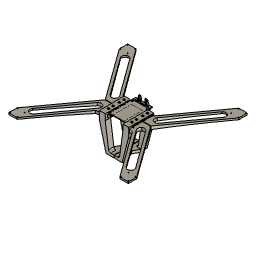
Drone Frame (Autodesk Fusion 360 design; units mm, degrees)
Autodesk Fusion 360 part; units mm, degrees
note: some values were not read from the file. Chosen so that the rebuilt part matches the saved one: a direction; which face or edge a step refers to. Set by a fixed rule: which sketch regions a step uses.
sketch "Sketch1" plane through (0, 0, 0) normal (0, 1, 0) x (1, 0, 0)
  line L0 (0, 0) -> (0, 2.5)
  line L1 (0, 0) -> (49.8, 0)
  line L2 (49.8, 0) -> (49.8, 2.5)
  line L3 (0, 2.5) -> (3, 2.5)
  line L4 (3, 2.5) -> (3, 7.5)
  line L5 (3, 7.5) -> (-2.5, 7.5)
  line L6 (-2.5, 7.5) -> (-2.5, -5)
  line L7 (-2.5, -5) -> (24.9, -5)
  line L8 (24.9, 0) -> (24.9, -5)
  line L9 (52.3, 7.5) -> (52.3, -5)
  line L10 (46.8, 7.5) -> (52.3, 7.5)
  line L11 (46.8, 2.5) -> (46.8, 7.5)
  line L12 (49.8, 2.5) -> (46.8, 2.5)
  line L13 (52.3, -5) -> (24.9, -5)
  dimension "d1" = 2.5
  dimension "d2" = 49.8
  dimension "d3" = 3
  dimension "d4" = 5
  dimension "d5" = 5
  dimension "d6" = 2.5
  constraint coincident L0.start L1.start
  constraint vertical L0
  constraint perpendicular L0 L1
  constraint perpendicular L1 L2
  constraint horizontal L0.end L2.end
  constraint perpendicular L0 L3
  constraint perpendicular L3 L4
  constraint perpendicular L4 L5
  constraint perpendicular L5 L6
  constraint perpendicular L6 L7
  constraint midpoint L1 L8.start
  constraint perpendicular L7 L8
  constraint symmetric L0.end L8 L2.end
  constraint symmetric L3.end L8 L11.start
  constraint symmetric L4.end L8 L10.start
  constraint symmetric L5.end L8 L9.start
  constraint symmetric L6.end L8 L9.end
  constraint symmetric L7.end L8 L13.end
  measures "d1" distance of L0.start L0.end
  measures "d2" distance of L0.start L1.end
  measures "d3" distance of L0.end L3.end
  measures "d4" distance of L3.end L4.end
  measures "d5" distance of L7.end L8.start
  measures "d6" distance of L0 L6
extrude "Extrude1" add sketch "Sketch1" along normal blind 65 makes body 1
sketch "Sketch2" plane through (0, 0, 0) normal (0, 0, -1) x (1, 0, 0)
  line L0 (49.8, 0) -> (0, 0)
  line L1 (0, 0) -> (0, -65)
  line L2 (0, -65) -> (49.8, -65)
  line L3 (49.8, -65) -> (49.8, 0)
  line L4 (49.8, -61) -> (0, -61)
  dimension "d9" = 4
  constraint coincident L3 L4.start
  constraint coincident L1 L4.end
  constraint perpendicular L1 L4
  measures "d9" distance of L2 L4
extrude "Extrude2" add sketch "Sketch2" along normal blind 4 contours L1 L2 L3 L4 bodies 1
sketch "Sketch3" plane through (0, 0, 0) normal (0, 0, -1) x (1, 0, 0)
  line L0 (0, -61) -> (49.8, -61)
  line L1 (49.8, -61) -> (49.8, 0)
  line L2 (49.8, 0) -> (0, 0)
  line L3 (0, 0) -> (0, -61)
  line L4 (3, 0) -> (3, -65)
  line L5 (46.8, 0) -> (46.8, -65)
  line L6 (46.8, -61) -> (3, -61)
  line L7 (0, 0) -> (49.8, 0)
  line L8 (3, -65) -> (46.8, -65)
  line L9 (46.8, -65) -> (46.8, 0)
  line L10 (46.8, 0) -> (3, 0)
  line L11 (3, 0) -> (3, -65)
  line L12 (3, -65) -> (3, -61)
  line L13 (46.8, -65) -> (46.8, -61)
  constraint horizontal L8
  constraint vertical L9
  constraint horizontal L10
  constraint vertical L11
  constraint coincident L5.start L9.end
  constraint coincident L4.end L8.start
extrude "Extrude3" cut sketch "Sketch3" against normal blind 5 contours L0 L4 L5 L6 L8 L9 L11 L12 L13 bodies 1
sketch "Sketch4" plane through (0, 0, 5) normal (0, 0, 1) x (-1, 0, 0)
  line L0 (-46.8, -65) -> (-46.8, -61)
  line L1 (-52.3, 0) -> (-52.3, -65)
  line L2 (-3, -65) -> (2.5, -65)
  line L3 (2.5, -65) -> (2.5, 0)
  line L4 (2.5, 0) -> (-52.3, 0)
  line L5 (-3, -61) -> (-3, -65)
  line L6 (-46.8, -61) -> (-3, -61)
  line L7 (-53.15, -65) -> (-53.15, -75)
  line L8 (-53.15, -75) -> (3.35, -75)
  line L9 (3.35, -75) -> (3.35, -65)
  line L10 (3.35, -65) -> (2.5, -65)
  line L11 (-52.3, -65) -> (-46.8, -65)
  line L12 (-53.15, -65) -> (-52.3, -65)
  dimension "d15" = 56.5
  dimension "d16" = 10
  constraint perpendicular L7 L8
  constraint perpendicular L8 L9
  constraint coincident L2.end L3.start
  constraint perpendicular L3 L10
  constraint coincident L1.end L11.start
  constraint horizontal L7.start L1.end
  constraint equal L10 L12
  constraint horizontal L8
  measures "d15" distance of L7.end L8.end
  measures "d16" distance of L7.start L7.end
extrude "Extrude4" add sketch "Sketch4" against normal blind 5 contours L0 L2 L5 L6 L7 L8 L9 L10 L11 L12 bodies 1
sketch "Sketch5" plane through (0, 0, 5) normal (0, 0, 1) x (-1, 0, 0)
  line L0 (-52.3, 0) -> (-52.3, -65)
  line L1 (-53.15, -65) -> (-53.15, -75)
  line L2 (-53.15, -75) -> (3.35, -75)
  line L3 (3.35, -75) -> (3.35, -65)
  line L4 (3.35, -65) -> (2.5, -65)
  line L5 (2.5, -65) -> (2.5, 0)
  line L6 (2.5, 0) -> (-52.3, 0)
  circle A0 centre (-0.4, -70) radius 1.4
  circle A1 centre (-49.4, -70) radius 1.4
  line L7 (-1.8, -70) -> (-48, -70)
  line L8 (-0.4, -70) -> (3.35, -70)
  line L9 (-49.4, -70) -> (-53.15, -70)
  line L10 (-52.3, -65) -> (-53.15, -65)
  dimension "d19" = 2.8
  dimension "d20" = 2.8
  dimension "d21" = 46.2
  dimension "d22" = 5
  constraint horizontal A0.centre A1.centre
  constraint coincident A0 L7.start
  constraint coincident A1 L7.end
  constraint horizontal L7
  constraint horizontal A1.centre L7.end
  constraint coincident A0.centre L8.start
  constraint coincident L3 L8.end
  constraint perpendicular L3 L8
  constraint coincident A1.centre L9.start
  constraint coincident L1 L9.end
  constraint perpendicular L1 L9
  constraint equal L8 L9
  measures "d19" diameter of A0
  measures "d20" diameter of A1
  measures "d21" distance of L7.start L7.end
  measures "d22" distance of L2 L7
extrude "Extrude5" cut sketch "Sketch5" against normal blind 8 contours A1 | A0 bodies 1
sketch "Sketch6" plane through (0, 0, 5) normal (0, 0, 1) x (-1, 0, 0)
  circle A0 centre (-49.4, -70) radius 1.4
  circle A1 centre (-0.4, -70) radius 1.4
  line L0 (-52.3, 0) -> (-52.3, -65)
  line L1 (-53.15, -65) -> (-53.15, -75)
  line L2 (-53.15, -75) -> (3.35, -75)
  line L3 (3.35, -75) -> (3.35, -65)
  line L4 (3.35, -65) -> (2.5, -65)
  line L5 (2.5, -65) -> (2.5, 0)
  line L6 (2.5, 0) -> (-52.3, 0)
  line L7 (-3, -61) -> (-46.8, -61)
  line L8 (-46.8, -61) -> (-46.8, -66)
  line L9 (-46.8, -66) -> (-3, -66)
  line L10 (-3, -66) -> (-3, -61)
  line L11 (-52.3, -65) -> (-53.15, -65)
  dimension "d25" = 5
  constraint horizontal L7
  constraint vertical L8
  constraint horizontal L9
  constraint vertical L10
  measures "d25" distance of L7.start L9.end
extrude "Extrude6" add sketch "Sketch6" against normal blind 2.5 contours L7 L8 L9 L10 bodies 1
sketch "Sketch7" plane through (0, 0, 5) normal (0, 0, 1) x (-1, 0, 0)
  line L0 (2.5, 0) -> (-52.3, 0)
  line L1 (-52.3, 0) -> (-52.3, -65)
  line L2 (-53.15, -65) -> (-53.15, -75)
  line L3 (-53.15, -75) -> (3.35, -75)
  line L4 (2.5, -65) -> (2.5, 0)
  line L5 (-52.3, 0) -> (-72.3, 0)
  line L6 (-72.3, 0) -> (-72.3, -65)
  line L7 (-72.3, -65) -> (-52.3, -65)
  line L8 (-52.3, -65) -> (-52.3, 0)
  line L9 (2.5, 0) -> (22.5, 0)
  line L10 (22.5, 0) -> (22.5, -65)
  line L11 (22.5, -65) -> (2.5, -65)
  line L12 (2.5, -65) -> (2.5, 0)
  line L13 (-52.3, -65) -> (-53.15, -65)
  dimension "d35" = 20
  dimension "d36" = 20
  constraint horizontal L5
  constraint vertical L6
  constraint horizontal L7
  constraint vertical L8
  constraint coincident L0.end L1.start
  constraint horizontal L9
  constraint vertical L10
  constraint horizontal L11
  constraint vertical L12
  constraint coincident L0.start L4.end
  constraint coincident L4.start L11.end
  constraint coincident L1.end L7
  measures "d35" distance of L6.end L1.end
  measures "d36" distance of L10.end L4.start
extrude "Extrude7" add sketch "Sketch7" against normal blind 12.5 bodies 1
sketch "Sketch8" plane through (-22.5, 0, 0) normal (-1, 0, 0) x (0, -1, 0)
  line L0 (-62.5, 2.75) -> (-2.5, 2.75)
  line L1 (-2.5, 2.75) -> (-2.5, -5.25)
  line L2 (-2.5, -5.25) -> (-62.5, -5.25)
  line L3 (-62.5, -5.25) -> (-62.5, 2.75)
  line L4 (0, 5) -> (-65, 5)
  line L5 (-65, 5) -> (-65, -4)
  line L6 (-65, -4) -> (0, -4)
  line L7 (0, -4) -> (0, 5)
  line L8 (0, 5) -> (-65, 5)
  line L9 (-65, 5) -> (-65, -7.5)
  line L10 (-65, -7.5) -> (0, -7.5)
  line L11 (0, -7.5) -> (0, 5)
  dimension "d104" = 60
  dimension "d105" = 8
  dimension "d106" = 2.5
  dimension "d126" = 2.25
  constraint horizontal L0
  constraint vertical L1
  constraint horizontal L2
  constraint vertical L3
  measures "d104" distance of L0.start L0.end
  measures "d105" distance of L0.start L2.end
  measures "d106" distance of L3 L5
  measures "d126" distance of L2 L10
extrude "Extrude8" cut sketch "Sketch8" against normal blind 20 contours L0 L1 L3 L6 | L1 L2 L3 L6 bodies 1
sketch "Sketch9" plane through (0, 0, 5) normal (0, 0, 1) x (-1, 0, 0)
  line L0 (22.5, 0) -> (-72.3, 0)
  line L1 (-72.3, 0) -> (-72.3, -65)
  line L2 (3.35, -65) -> (22.5, -65)
  line L3 (-53.15, -65) -> (-53.15, -75)
  line L4 (-53.15, -75) -> (3.35, -75)
  line L5 (3.35, -75) -> (3.35, -65)
  line L6 (22.5, -65) -> (22.5, 0)
  circle A0 centre (-49.4, -70) radius 1.4
  circle A1 centre (-0.4, -70) radius 1.4
  circle A2 centre (12.75, -57.5) radius 2.5
  circle A3 centre (12.75, -7.5) radius 2.5
  circle A4 centre (12.75, -22.5) radius 2.5
  circle A5 centre (12.75, -42.5) radius 2.5
  line L7 (-24.9, 0) -> (-24.9, -61)
  circle A6 centre (-62.55, -57.5) radius 2.5
  circle A7 centre (-62.55, -42.5) radius 2.5
  circle A8 centre (-62.55, -22.5) radius 2.5
  circle A9 centre (-62.55, -7.5) radius 2.5
  line L8 (-72.3, -65) -> (-53.15, -65)
  dimension "d56" = 5
  dimension "d60" = 5
  dimension "d62" = 7.5
  dimension "d116" = 9.75
  dimension "d117" = 7.5
  dimension "d120" = 0
  dimension "d121" = -15
  dimension "d124" = 0
  dimension "d125" = 15
  constraint vertical A2.centre A3.centre
  constraint midpoint L0 L7.start
  constraint symmetric A2 L7 A6
  constraint symmetric A3 L7 A9
  constraint symmetric A4 L7 A8
  constraint symmetric A5 L7 A7
  measures "d56" diameter of A2
  measures "d60" diameter of A3
  measures "d62" vertical distance of L0.start A3.centre
  measures "d116" distance of L6 A2.centre
  measures "d117" vertical distance of L2.end A2.centre
extrude "Extrude10" cut sketch "Sketch9" against normal through all contours A2 | A3 | A4 | A5 | A6 | A7 | A8 | A9 bodies 1
chamfer "Chamfer1" distance 1 angle 45 8 edges at (-10.4192, 56.596, 5) (-10.4192, 6.596, 5) (-10.4192, 21.596, 5) (-10.4192, 41.596, 5) (64.8808, 56.596, 5) (64.8808, 41.596, 5) (64.8808, 21.596, 5) (64.8808, 6.596, 5) on bodies 1
ref_plane "WorkPlane1" through (24.9, 37.5, 2.75) normal (0, 0, 1) x (1, 0, 0)
sketch "Sketch10" plane through (0, 0, 2.75) normal (0, 0, 1) x (1, 0, 0)
  line L0 (-2.75, 2.75) -> (-23, 2.75)
  line L1 (-23, 2.75) -> (-140.5571, -159.0534)
  line L2 (-140.5571, -159.0534) -> (-167.6747, -159.0534)
  line L3 (-167.6747, -159.0534) -> (-167.6747, -131.9358)
  line L4 (-23, 2.75) -> (-69.8197, 2.75)
  line L5 (-22.75, 31.75) -> (-48.75, 31.75)
  line L6 (-48.75, 31.75) -> (-167.6747, -131.9358)
  line L7 (-22.75, 31.75) -> (-2.75, 31.75)
  line L8 (-22.5, 65) -> (-3.35, 65)
  line L9 (-2.75, 2.75) -> (-2.75, 31.75)
  line L10 (72.3, 0) -> (-22.5, 0)
  line L11 (-2.5, 62.5) -> (-2.5, 2.5)
  line L12 (-2.5, 2.5) -> (-2.5, 62.5)
  line L13 (-23, 2.75) -> (-23, 31.75)
  dimension "d77" = 54
  dimension "d79" = 26
  dimension "d86" = 20
  dimension "d98" = 200
  dimension "d112" = 0.25
  dimension "d113" = 29
  dimension "d114" = 0.25
  dimension "d115" = 20.25
  constraint perpendicular L2 L3
  constraint horizontal L2
  constraint parallel L1 L6
  constraint equal L2 L3
  constraint coincident L4.end L6
  constraint vertical L9
  constraint horizontal L5
  constraint horizontal L7
  constraint horizontal L0
  constraint horizontal L4
  constraint coincident L0.start L9.start
  constraint coincident L5 L13.end
  constraint perpendicular L5 L13
  measures "d77" angle of L1 L4
  measures "d79" distance of L5.start L5.end
  measures "d86" distance of L5.start L7.end
  measures "d98" distance of L0.end L1.end
  measures "d112" vertical distance of L0.start L11.end
  measures "d113" distance of L0.start L7.end
  measures "d114" distance of L9 L11
  measures "d115" distance of L0.start L0.end
extrude "Extrude11" add sketch "Sketch10" against normal blind 7.8 separate body contours L0 L5 L7 L9 L13 makes body 2
extrude "Extrude12" add sketch "Sketch10" against normal blind 10 contours L1 L2 L3 L4 L6 | L4 L5 L6 L13 bodies 2
sketch "Sketch11" plane through (0, 0, 2.75) normal (0, 0, 1) x (-1, 0, 0)
  line L0 (2.75, -31.75) -> (48.75, -31.75)
  line L1 (48.75, -31.75) -> (167.6747, 131.9358)
  line L2 (167.6747, 131.9358) -> (167.6747, 159.0534)
  line L3 (167.6747, 159.0534) -> (140.5571, 159.0534)
  line L4 (140.5571, 159.0534) -> (23, -2.75)
  line L5 (23, -2.75) -> (2.75, -2.75)
  line L6 (29.2805, -7.716) -> (123.3261, 121.7267)
  line L7 (46.9801, -20.5756) -> (29.2805, -7.716)
  line L8 (2.75, -2.75) -> (2.75, -31.75)
  arc A0 (141.0258, 108.8671) -> (123.3261, 121.7267) centre (132.176, 115.2969) ccw
  line L9 (46.9801, -20.5756) -> (141.0258, 108.8671)
  dimension "d89" = 8
  dimension "d90" = 8
  dimension "d136" = 8
  dimension "d137" = 160
  constraint parallel L4 L6
  constraint perpendicular L6 L7
  constraint tangent L6 A0
  constraint tangent A0 L9
  constraint parallel L6 L9
  measures "d89" distance of L4 L6
  measures "d90" distance of L0.end L7
  measures "d136" distance of L1 L9
  measures "d137" distance of A0.start L7.start
extrude "Extrude13" cut sketch "Sketch11" against normal blind 10 contours L6 L7 A0 L9 bodies 2
sketch "Sketch12" plane through (0, 0, 2.75) normal (0, 0, 1) x (-1, 0, 0)
  line L0 (46.9801, -20.5756) -> (29.2805, -7.716)
  line L1 (29.2805, -7.716) -> (123.3261, 121.7267)
  line L2 (2.75, -31.75) -> (48.75, -31.75)
  line L3 (48.75, -31.75) -> (167.6747, 131.9358)
  line L4 (167.6747, 131.9358) -> (167.6747, 159.0534)
  line L5 (167.6747, 159.0534) -> (140.5571, 159.0534)
  line L6 (140.5571, 159.0534) -> (23, -2.75)
  line L7 (23, -2.75) -> (2.75, -2.75)
  circle A0 centre (165.1747, 156.5534) radius 1.55
  circle A1 centre (141.8402, 156.5534) radius 1.55
  circle A2 centre (141.8402, 133.2189) radius 1.55
  circle A3 centre (165.1747, 133.2189) radius 1.55
  line L8 (165.1747, 133.2189) -> (141.8402, 133.2189)
  line L9 (141.8402, 133.2189) -> (141.8402, 156.5534)
  line L10 (141.8402, 156.5534) -> (165.1747, 156.5534)
  line L11 (165.1747, 156.5534) -> (167.6747, 156.5534)
  line L12 (141.8402, 156.5534) -> (141.8402, 159.0534)
  line L13 (2.75, -2.75) -> (2.75, -31.75)
  line L14 (141.0258, 108.8671) -> (46.9801, -20.5756)
  arc A4 (141.0258, 108.8671) -> (123.3261, 121.7267) centre (132.176, 115.2969) ccw
  dimension "d95" = 3.1
  dimension "d97" = 33
  dimension "d99" = 2.5
  constraint equal A0 A3
  constraint equal A0 A1
  constraint equal A1 A2
  constraint vertical A1.centre A2.centre
  constraint horizontal A0.centre A1.centre
  constraint vertical A0.centre A3.centre
  constraint horizontal A2.centre A3.centre
  constraint coincident A3.centre L8.start
  constraint coincident A2.centre L8.end
  constraint coincident A1.centre L9.end
  constraint coincident A0.centre L10.end
  constraint equal L9 L10
  constraint coincident L4 L11.end
  constraint perpendicular L4 L11
  constraint coincident L5 L12.end
  constraint perpendicular L5 L12
  constraint equal L11 L12
  measures "d95" diameter of A0
  measures "d97" distance of A1.centre A3.centre
  measures "d99" distance of A0.centre L11.end
extrude "Extrude14" cut sketch "Sketch12" against normal through all contours A0 L10 L11 | A0 L10 L11 | A1 L9 L12 | A1 L10 L12 | A1 L9 L10 | A2 L8 L9 | A2 L8 L9 | A3 bodies 2
sketch "Sketch13" plane through (-47.0053, 34.1514, 0) normal (-0.809017, 0.587785, 0) x (-0.587785, -0.809017, 0)
  line L0 (205.295, 2.75) -> (2.9682, 2.75)
  line L1 (2.9682, 2.75) -> (2.9682, -7.25)
  line L2 (2.9682, -7.25) -> (205.295, -7.25)
  line L3 (205.295, -7.25) -> (205.295, 2.75)
  line L4 (181.9072, 2.75) -> (181.9072, -7.25)
  line L5 (227.2336, 2.75) -> (227.2336, -7.25)
  line L6 (181.9072, -2.25) -> (227.2336, -2.25)
  line L7 (227.2336, -7.25) -> (205.295, -7.25)
  arc A0 (181.9072, -2.25) -> (2.9682, -7.25) centre (181.9072, -3206.6659) ccw
  line L8 (170.9682, 2.75) -> (181.9072, 2.75)
  point P0 (181.9072, 2.75)
  constraint coincident L0 P0
  constraint coincident L2 L4.end
  constraint perpendicular L2 L4
  constraint coincident P0 L4.start
  constraint midpoint L6.start L4
  constraint midpoint L5 L6.end
  constraint coincident L5.end L7.start
  constraint coincident L2.end L3.start
  constraint coincident L1.end L2.start
  constraint tangent L6 A0
extrude "Extrude15" cut sketch "Sketch13" against normal blind 100 contours L3 L5 L6 L7 | L2 L3 L4 L6 | L2 L4 A0 bodies 2
extrude "Extrude16" cut sketch "Sketch8" along normal blind 20 from surface at -94.8 contours L0 L1 L3 L6 | L1 L2 L3 L6 bodies 1
fillet "Fillet1" radius 4 2 edges at (3, 32.5, -7.5) (46.8, 32.5, -7.5) on bodies 1
sketch "Sketch14" plane through (0, 0, 2.75) normal (0, 0, 1) x (-1, 0, 0)
  circle A0 centre (165.1747, 133.2189) radius 1.55
  circle A1 centre (141.8402, 156.5534) radius 1.55
  circle A2 centre (165.1747, 156.5534) radius 1.55
  line L0 (46.9801, -20.5756) -> (29.2805, -7.716)
  line L1 (29.2805, -7.716) -> (123.3261, 121.7267)
  line L2 (2.75, -2.75) -> (2.75, -31.75)
  line L3 (2.75, -31.75) -> (48.75, -31.75)
  line L4 (48.75, -31.75) -> (167.6747, 131.9358)
  line L5 (167.6747, 131.9358) -> (167.6747, 159.0534)
  line L6 (167.6747, 159.0534) -> (140.5571, 159.0534)
  line L7 (140.5571, 159.0534) -> (23, -2.75)
  line L8 (23, -2.75) -> (2.75, -2.75)
  circle A3 centre (12.75, -7.5) radius 2.5
  circle A4 centre (12.75, -22.5) radius 2.5
  line L9 (141.0258, 108.8671) -> (46.9801, -20.5756)
  arc A5 (141.0258, 108.8671) -> (123.3261, 121.7267) centre (132.176, 115.2969) ccw
  circle A6 centre (141.8402, 133.2189) radius 1.55
extrude "Extrude17" cut sketch "Sketch14" against normal blind 15 contours A3 | A4 bodies 1 2
fillet "Fillet2" radius 11 2 edges at (-46.9801, 20.5756, -2.0313) (-29.2805, 7.716, -2.0313) on bodies 2
copy_body "CopyPasteBodies1" bodies 2 makes body 3
move_body "Move1" bodies 3 to x (-1, 0, 0) y (0, -1, 0) z (0, 0, 1) at (-5.5, 63.5, 0)
move_body "Align1" bodies 3 to x (1, 0, 0) y (0, 1, 0) z (0, 0, 1) at (55.3, 1.5, 1.25)
sketch "Sketch15" plane through (0, 0, 2.75) normal (0, 0, 1) x (-1, 0, 0)
  circle A0 centre (12.75, -7.5) radius 2.5
  circle A1 centre (12.75, -22.5) radius 2.5
  circle A2 centre (141.8402, 133.2189) radius 1.55
  circle A3 centre (165.1747, 133.2189) radius 1.55
  circle A4 centre (141.8402, 156.5534) radius 1.55
  circle A5 centre (165.1747, 156.5534) radius 1.55
  line L0 (141.0258, 108.8671) -> (53.4458, -11.6764)
  arc A6 (38.081, -14.1099) -> (53.4458, -11.6764) centre (44.5466, -5.2108) ccw
  arc A7 (35.7457, 1.1826) -> (38.081, -14.1099) centre (44.6449, -5.283) ccw
  line L1 (35.7457, 1.1826) -> (123.3261, 121.7267)
  arc A8 (141.0258, 108.8671) -> (123.3261, 121.7267) centre (132.176, 115.2969) ccw
  line L2 (2.75, -2.75) -> (2.75, -31.75)
  line L3 (2.75, -31.75) -> (48.75, -31.75)
  line L4 (48.75, -31.75) -> (167.6747, 131.9358)
  line L5 (167.6747, 131.9358) -> (167.6747, 159.0534)
  line L6 (167.6747, 159.0534) -> (140.5571, 159.0534)
  line L7 (140.5571, 159.0534) -> (23, -2.75)
  line L8 (23, -2.75) -> (2.75, -2.75)
  line L9 (165.1747, 133.2189) -> (141.8402, 156.5534)
  circle A9 centre (-62.55, -57.5) radius 2.5
  circle A10 centre (-62.55, -42.5) radius 2.5
  circle A11 centre (-191.6402, -198.2189) radius 1.55
  circle A12 centre (-214.9747, -198.2189) radius 1.55
  circle A13 centre (-191.6402, -221.5534) radius 1.55
  circle A14 centre (-214.9747, -221.5534) radius 1.55
  line L10 (-190.8258, -173.8671) -> (-103.2458, -53.3236)
  arc A15 (-87.881, -50.8901) -> (-103.2458, -53.3236) centre (-94.3466, -59.7892) ccw
  arc A16 (-85.5457, -66.1826) -> (-87.881, -50.8901) centre (-94.4449, -59.717) ccw
  line L11 (-85.5457, -66.1826) -> (-173.1261, -186.7267)
  arc A17 (-190.8258, -173.8671) -> (-173.1261, -186.7267) centre (-181.976, -180.2969) ccw
  line L12 (-52.55, -62.25) -> (-52.55, -33.25)
  line L13 (-52.55, -33.25) -> (-98.55, -33.25)
  line L14 (-98.55, -33.25) -> (-217.4747, -196.9358)
  line L15 (-217.4747, -196.9358) -> (-217.4747, -224.0534)
  line L16 (-217.4747, -224.0534) -> (-190.3571, -224.0534)
  line L17 (-190.3571, -224.0534) -> (-72.8, -62.25)
  line L18 (-72.8, -62.25) -> (-52.55, -62.25)
  line L19 (-191.6402, -221.5534) -> (-214.9747, -198.2189)
  line L20 (165.1747, 156.5534) -> (153.5074, 144.8861)
  line L21 (-214.9747, -221.5534) -> (-203.3074, -209.8861)
  constraint coincident A3.centre L9.start
  constraint coincident A4.centre L9.end
  constraint coincident A13.centre L19.start
  constraint coincident A12.centre L19.end
  constraint coincident A5.centre L20.start
  constraint midpoint L9 L20.end
  constraint coincident A14.centre L21.start
  constraint midpoint L19 L21.end
sketch "Sketch16" plane through (0, 0, 5) normal (0, 0, 1) x (-1, 0, 0)
  circle A0 centre (-62.55, -22.5) radius 3.5
  circle A1 centre (-62.55, -57.5) radius 3.5
  circle A2 centre (12.75, -22.5) radius 3.5
  circle A3 centre (12.75, -57.5) radius 3.5
  circle A4 centre (-49.4, -70) radius 1.4
  circle A5 centre (-0.4, -70) radius 1.4
  line L0 (-53.15, -65) -> (-53.15, -75)
  line L1 (-53.15, -75) -> (3.35, -75)
  line L2 (3.35, -75) -> (3.35, -65)
  line L3 (3.35, -65) -> (22.5, -65)
  line L4 (22.5, -65) -> (22.5, 0)
  line L5 (22.5, 0) -> (-72.3, 0)
  line L6 (-72.3, 0) -> (-72.3, -65)
  line L7 (-72.3, -65) -> (-53.15, -65)
  circle A6 centre (12.75, -7.5) radius 3.5
  circle A7 centre (12.75, -42.5) radius 3.5
  circle A8 centre (-62.55, -42.5) radius 3.5
  circle A9 centre (-62.55, -7.5) radius 3.5
  line L8 (-24.9, -75) -> (-24.9, 0)
  constraint midpoint L1 L8.start
  constraint midpoint L5 L8.end
ref_plane "WorkPlane2" through (24.9, 37.5, 5) normal (-1, 0, 0) x (0, -1, 0)
mirror "Mirror1" about plane through (24.9, 37.5, 5) normal (-1, 0, 0) of bodies 2 3 makes body 4 at (199.8363, -148.4715, 2.75) makes body 5 at (-156.9785, 206.3007, 4)
sketch "Sketch17" plane through (0, 0, 0) normal (0, -1, 0) x (1, 0, 0)
  line L0 (50.8, -7.5) -> (72.3, -7.5)
  line L1 (72.3, -7.5) -> (72.3, 5)
  line L2 (72.3, 5) -> (-22.5, 5)
  line L3 (-22.5, 5) -> (-22.5, -7.5)
  line L4 (-22.5, -7.5) -> (-1, -7.5)
  line L5 (0, 0) -> (3, 0)
  line L6 (3, 0) -> (3, 3)
  line L7 (3, 3) -> (46.8, 3)
  line L8 (46.8, 3) -> (46.8, 0)
  line L9 (46.8, 0) -> (49.8, 0)
  line L10 (49.8, 0) -> (49.8, -2.5)
  line L11 (0, 0) -> (49.8, 0)
  point P0 (3, -2.5)
  dimension "d147" = 3
  constraint coincident L5.start L11.start
  constraint horizontal L5
  constraint perpendicular L5 L6
  constraint perpendicular L6 L7
  constraint coincident L9.end L10
  constraint coincident L9.end L10.start
  constraint coincident L8.end L11
  constraint vertical L8
  constraint equal L5 L9
  constraint vertical L5.end P0
  measures "d147" distance of L5.end L6.end
extrude "Extrude18" cut sketch "Sketch17" against normal blind 61 bodies 1
fillet "Fillet3" radius 5 2 edges at (3, 30.5, 3) (46.8, 30.5, 3) on bodies 1
sketch "Sketch18" plane through (0, 0, 2.75) normal (0, 0, 1) x (-1, 0, 0)
  circle A0 centre (12.75, -7.5) radius 2.5
  circle A1 centre (12.75, -22.5) radius 2.5
  circle A2 centre (141.8402, 133.2189) radius 1.55
  circle A3 centre (165.1747, 133.2189) radius 1.55
  circle A4 centre (141.8402, 156.5534) radius 1.55
  circle A5 centre (165.1747, 156.5534) radius 1.55
  line L0 (141.0258, 108.8671) -> (53.4458, -11.6764)
  arc A6 (38.081, -14.1099) -> (53.4458, -11.6764) centre (44.5466, -5.2108) ccw
  arc A7 (35.7457, 1.1826) -> (38.081, -14.1099) centre (44.6449, -5.283) ccw
  line L1 (35.7457, 1.1826) -> (123.3261, 121.7267)
  arc A8 (141.0258, 108.8671) -> (123.3261, 121.7267) centre (132.176, 115.2969) ccw
  line L2 (2.75, -2.75) -> (2.75, -31.75)
  line L3 (2.75, -31.75) -> (48.75, -31.75)
  line L4 (48.75, -31.75) -> (167.6747, 131.9358)
  line L5 (167.6747, 131.9358) -> (167.6747, 159.0534)
  line L6 (167.6747, 159.0534) -> (140.5571, 159.0534)
  line L7 (140.5571, 159.0534) -> (23, -2.75)
  line L8 (23, -2.75) -> (2.75, -2.75)
  line L9 (25.1796, 0.25) -> (-3, 0.25)
  line L10 (-3, 0.25) -> (-3, 3)
  line L11 (-3, 3) -> (34.4727, 13.0408)
  point P0 (-3, 0)
  point P1 (-46.8, 0)
  dimension "d150" = 0.25
  dimension "d151" = 105
  dimension "d152" = 2.75
  constraint coincident L7 L9.start
  constraint horizontal L9
  constraint vertical L9.end P0
  constraint perpendicular L9 L10
  constraint coincident L7 L11.end
  measures "d150" distance of L9 P0
  measures "d151" angle of L10 L11
  measures "d152" distance of L9.end L10.end
extrude "Extrude19" add sketch "Sketch18" against normal blind 8.5 contours L7 L9 L10 L11 bodies 2
sketch "Sketch19" plane through (0, 0, 2.75) normal (0, 0, 1) x (-1, 0, 0)
  circle A0 centre (-62.55, -7.5) radius 2.5
  circle A1 centre (-62.55, -22.5) radius 2.5
  circle A2 centre (-191.6402, 133.2189) radius 1.55
  circle A3 centre (-214.9747, 133.2189) radius 1.55
  circle A4 centre (-191.6402, 156.5534) radius 1.55
  circle A5 centre (-214.9747, 156.5534) radius 1.55
  line L0 (-103.2458, -11.6764) -> (-190.8258, 108.8671)
  arc A6 (-173.1261, 121.7267) -> (-190.8258, 108.8671) centre (-181.976, 115.2969) ccw
  line L1 (-173.1261, 121.7267) -> (-85.5457, 1.1826)
  arc A7 (-87.881, -14.1099) -> (-85.5457, 1.1826) centre (-94.4449, -5.283) ccw
  arc A8 (-103.2458, -11.6764) -> (-87.881, -14.1099) centre (-94.3466, -5.2108) ccw
  line L2 (-52.55, -31.75) -> (-52.55, -2.75)
  line L3 (-52.55, -2.75) -> (-72.8, -2.75)
  line L4 (-72.8, -2.75) -> (-190.3571, 159.0534)
  line L5 (-190.3571, 159.0534) -> (-217.4747, 159.0534)
  line L6 (-217.4747, 159.0534) -> (-217.4747, 131.9358)
  line L7 (-217.4747, 131.9358) -> (-98.55, -31.75)
  line L8 (-98.55, -31.75) -> (-52.55, -31.75)
  line L9 (-74.9796, 0.25) -> (-46.8, 0.25)
  line L10 (-46.8, 0.25) -> (-46.8, 3)
  line L11 (-46.8, 3) -> (-84.2727, 13.0408)
  point P0 (-46.8, 0)
  dimension "d157" = 0.25
  dimension "d158" = 2.75
  dimension "d159" = 105
  constraint coincident L4 L9.start
  constraint horizontal L9
  constraint vertical L9.end P0
  constraint perpendicular L9 L10
  constraint coincident L4 L11.end
  measures "d157" distance of L9.end P0
  measures "d158" distance of L9.end L10.end
  measures "d159" angle of L10 L11
extrude "Extrude20" add sketch "Sketch19" against normal blind 8.5 contours L4 L9 L10 L11 bodies 4
fillet "Fillet4" radius 3 2 edges at (3, -1.625, -5.75) (46.8, -1.625, -5.75) on bodies 2 4
sketch "Sketch20" plane through (0, 0, 5) normal (0, 0, 1) x (-1, 0, 0)
  circle A0 centre (-62.55, -22.5) radius 3.5
  circle A1 centre (-62.55, -57.5) radius 3.5
  circle A2 centre (12.75, -22.5) radius 3.5
  circle A3 centre (12.75, -57.5) radius 3.5
  circle A4 centre (-49.4, -70) radius 1.4
  circle A5 centre (-0.4, -70) radius 1.4
  line L0 (-53.15, -65) -> (-53.15, -75)
  line L1 (-53.15, -75) -> (3.35, -75)
  line L2 (3.35, -75) -> (3.35, -65)
  line L3 (3.35, -65) -> (22.5, -65)
  line L4 (22.5, -65) -> (22.5, 0)
  line L5 (22.5, 0) -> (-72.3, 0)
  line L6 (-72.3, 0) -> (-72.3, -65)
  line L7 (-72.3, -65) -> (-53.15, -65)
  circle A6 centre (12.75, -7.5) radius 3.5
  circle A7 centre (12.75, -42.5) radius 3.5
  circle A8 centre (-62.55, -42.5) radius 3.5
  circle A9 centre (-62.55, -7.5) radius 3.5
  circle A10 centre (-49.4, -70) radius 2.5
  circle A11 centre (-0.4, -70) radius 2.5
  line L8 (-51.9, -70) -> (-51.9, -78)
  line L9 (2.1, -70) -> (2.1, -78)
  line L10 (-46.9, -70) -> (-46.9, -78)
  line L11 (-2.9, -70) -> (-2.9, -78)
  line L12 (-51.9, -78) -> (-51.9, -84)
  line L13 (-51.9, -84) -> (2.1, -84)
  line L14 (2.1, -84) -> (2.1, -78)
  line L15 (-2.9, -78) -> (-46.9, -78)
  dimension "d162" = 5
  dimension "d163" = 6
  dimension "d165" = 3
  constraint concentric A4 A10
  constraint concentric A5 A11
  constraint equal A10 A11
  constraint coincident A10 L8.start
  constraint perpendicular L1 L8
  constraint tangent A10 L8
  constraint coincident A11 L9.start
  constraint perpendicular L1 L9
  constraint tangent A11 L9
  constraint horizontal L8.end L9.end
  constraint coincident A10 L10.start
  constraint tangent A10 L10
  constraint horizontal L8.end L10.end
  constraint vertical L10
  constraint coincident A11 L11.start
  constraint vertical L11
  constraint tangent A11 L11
  constraint horizontal L9.end L11.end
  constraint perpendicular L1 L12
  constraint perpendicular L8 L13
  constraint vertical L14
  measures "d162" diameter of A10
  measures "d163" distance of L9.end L13.end
  measures "d165" distance of L1 L15
extrude "Extrude21" add sketch "Sketch20" along normal blind 2 separate body contours L1 A10 L8 L10 | L1 L8 L9 L10 L11 L12 L13 L14 L15 | A10 | L1 A11 L9 L11 | A11 makes body 6
sketch "Sketch21" plane through (0, 0, 7) normal (0, 0, 1) x (-1, 0, 0)
  circle A0 centre (-0.4, -70) radius 1.4
  circle A1 centre (-49.4, -70) radius 1.4
  arc A2 (2.1, -70) -> (-2.9, -70) centre (-0.4, -70) ccw
  line L0 (-2.9, -70) -> (-2.9, -78)
  line L1 (-2.9, -78) -> (-46.9, -78)
  line L2 (-46.9, -78) -> (-46.9, -70)
  arc A3 (-46.9, -70) -> (-51.9, -70) centre (-49.4, -70) ccw
  line L3 (-51.9, -70) -> (-51.9, -84)
  line L4 (-51.9, -84) -> (2.1, -84)
  line L5 (2.1, -84) -> (2.1, -70)
  line L6 (-12.4, -80) -> (-12.4, -81.1)
  line L7 (-12.4, -81.1) -> (-37.4, -81.1)
  line L8 (-37.4, -81.1) -> (-37.4, -80)
  line L9 (-37.4, -80) -> (-51.9, -80)
  line L10 (-12.4, -80) -> (2.1, -80)
  line L11 (-38.4, -80) -> (-38.4, -82.1)
  line L12 (-38.4, -82.1) -> (-31.4, -82.1)
  line L13 (-31.4, -82.1) -> (-31.4, -81.1)
  line L14 (-38.4, -80) -> (-38.4, -79)
  line L15 (-38.4, -79) -> (-34.9, -79)
  line L16 (-34.9, -79) -> (-34.9, -80)
  line L17 (-34.9, -80) -> (-37.4, -80)
  line L18 (-11.4, -80) -> (-11.4, -82.1)
  line L19 (-11.4, -82.1) -> (-17.4, -82.1)
  line L20 (-17.4, -82.1) -> (-17.4, -81.1)
  line L21 (-11.4, -80) -> (-11.4, -79)
  line L22 (-11.4, -79) -> (-16.4, -79)
  line L23 (-16.4, -79) -> (-16.4, -80)
  line L24 (-16.4, -80) -> (-12.4, -80)
  dimension "d169" = 25
  dimension "d170" = 1.1
  dimension "d171" = 1
  dimension "d172" = 6
  dimension "d173" = 4
  dimension "d175" = 1
  dimension "d176" = 2.5
  dimension "d177" = 1
  dimension "d178" = 1
  dimension "d179" = 1
  dimension "d180" = 6
  dimension "d181" = 4
  dimension "d182" = 1
  constraint vertical L6
  constraint horizontal L7
  constraint vertical L8
  constraint coincident L3 L9.end
  constraint perpendicular L3 L9
  constraint coincident L5 L10.end
  constraint perpendicular L5 L10
  constraint equal L9 L10
  constraint coincident L9 L11.start
  constraint perpendicular L9 L11
  constraint perpendicular L11 L12
  constraint coincident L7 L13.end
  constraint perpendicular L7 L13
  constraint perpendicular L9 L14
  constraint perpendicular L11 L15
  constraint perpendicular L15 L16
  constraint perpendicular L8 L17
  constraint coincident L10 L18.start
  constraint perpendicular L10 L18
  constraint perpendicular L18 L19
  constraint coincident L7 L20.end
  constraint perpendicular L7 L20
  constraint perpendicular L10 L21
  constraint perpendicular L21 L22
  constraint perpendicular L22 L23
  constraint perpendicular L6 L24
  constraint horizontal L15.end L22.end
  measures "d169" distance of L8.end L6.start
  measures "d170" distance of L8.end L7.end
  measures "d171" distance of L8 L11
  measures "d172" distance of L7.end L13.end
  measures "d173" distance of L3.end L9.end
  measures "d175" distance of L12.end L13.end
  measures "d176" distance of L8.end L16
  measures "d177" distance of L11.start L14.end
  measures "d178" distance of L7 L19.end
  measures "d179" distance of L6 L18
  measures "d180" distance of L18.end L19.end
  measures "d181" distance of L6.start L23.end
  measures "d182" distance of L22.end L23.end
extrude "Extrude22" add sketch "Sketch21" along normal blind 15 contours L6 L7 L10 L18 L19 L20 | L9 L14 L15 L16 L17 | L7 L8 L9 L11 L12 L13 bodies 6
extrude "Extrude23" add sketch "Sketch21" along normal blind 4 contours L10 L21 L22 L23 L24 bodies 6
chamfer "Chamfer2" distance 1.9 distance2 15 2 edges at (34.9, 82.1, 7) (14.4, 82.1, 7) measured on face at (45.7333, 81.3667, 7) measured on face at (45.7333, 81.3667, 7) on bodies 6
chamfer "Chamfer3" distance 3 distance2 15 2 edges at (38.4, 81.5, 7) (11.4, 81.5, 7) measured on face at (45.7333, 81.9999, 7) measured on face at (45.7333, 81.9999, 7) on bodies 6
sketch "Sketch22" plane through (24.9, 0, 0) normal (-1, 0, 0) x (0, -1, 0)
  line L0 (-2.4, 9) -> (-2.4, 26.9)
  line L1 (-2.4, 26.9) -> (-3.5, 28)
  line L2 (-3.5, 28) -> (0, 28)
  line L3 (0, 28) -> (0, 9)
  line L4 (0, 9) -> (-2.4, 9)
  dimension "d191" = 45
  dimension "d192" = 2.4
  dimension "d193" = 3.5
  dimension "d194" = 9
  dimension "d195" = 19
  constraint horizontal L2
  constraint vertical origin L3.end
  constraint perpendicular L0 L4
  constraint vertical L3
  constraint vertical L0
  measures "d191" angle of L1 L2
  measures "d192" distance of L0.start L3.end
  measures "d193" distance of L1.end L2.end
  measures "d194" distance of origin L3.end
  measures "d195" distance of L2.end L3.end
revolve "Revolve1" add sketch "Sketch22" angle 360 about axis through (24.9, 0, 28) along (0, 0, -1) separate body makes body 7
chamfer "Chamfer4" distance 0.8 angle 45 1 edges at (22.6624, -0.8679, 9) on bodies 7
move_body "Align2" bodies 7 to x (1, 0, 0) y (0, 1, 0) z (0, 0, 1) at (-37.65, 7.5, -23)
sketch "Sketch23" plane through (72.3, 0, 0) normal (1, 0, 0) x (0, 1, 0)
  line L0 (62.5, -5.25) -> (2.5, -5.25)
  line L1 (2.5, -5.25) -> (2.5, 2.75)
  line L2 (2.5, 2.75) -> (62.5, 2.75)
  line L3 (62.5, 2.75) -> (62.5, -5.25)
  line L4 (65, 5) -> (0, 5)
  line L5 (0, 5) -> (0, -7.5)
  line L6 (0, -7.5) -> (65, -7.5)
  line L7 (65, -7.5) -> (65, 5)
  line L8 (-12.25, 8.25) -> (-12.25, -10.75)
  line L9 (-12.25, -10.75) -> (68.25, -10.75)
  line L10 (68.25, -10.75) -> (68.25, 8.25)
  line L11 (68.25, 8.25) -> (-12.25, 8.25)
  line L12 (-0.25, 5.25) -> (65.25, 5.25)
  line L13 (65.25, 5.25) -> (65.25, -7.75)
  line L14 (65.25, -7.75) -> (-0.25, -7.75)
  line L15 (-0.25, -7.75) -> (-0.25, 5.25)
  dimension "d198" = 0.25
  dimension "d199" = 0.25
  dimension "d200" = 0.25
  dimension "d201" = 12
  dimension "d202" = 3
  dimension "d203" = 3
  dimension "d204" = 3
  dimension "d205" = 0.25
  constraint perpendicular L4 L8
  constraint perpendicular L5 L9
  constraint perpendicular L9 L10
  constraint horizontal L11
  constraint horizontal L12
  constraint vertical L13
  constraint horizontal L14
  constraint vertical L15
  measures "d198" distance of L6 L14
  measures "d199" distance of L4 L12
  measures "d200" distance of L7 L13
  measures "d201" distance of L8 L15
  measures "d202" distance of L9 L14
  measures "d203" distance of L11 L12
  measures "d204" distance of L10 L13
  measures "d205" distance of L5 L15
extrude "Extrude24" add sketch "Sketch23" against normal blind 19 separate body contours L8 L9 L10 L11 makes body 8
sketch "Sketch24" plane through (0, 68.25, 0) normal (0, 1, 0) x (-1, 0, 0)
  line L0 (-72.3, 8.25) -> (-72.3, -10.75)
  line L1 (-72.3, -10.75) -> (-53.3, -10.75)
  line L2 (-53.3, -10.75) -> (-53.3, 8.25)
  line L3 (-53.3, 8.25) -> (-72.3, 8.25)
  line L4 (-50.6513, -100.75) -> (-40.6513, -100.75)
  line L5 (-40.6513, -100.75) -> (-53.3, -10.75)
  arc A0 (-72.3, -10.75) -> (-70.7046, -23.2796) centre (-22.3, -10.75) ccw
  line L6 (-70.7046, -23.2796) -> (-50.6513, -100.75)
  dimension "d210" = 10
  dimension "d216" = 50
  dimension "d228" = 98
  dimension "d232" = 90
  constraint perpendicular L0 L4
  constraint coincident L1.end L2.start
  constraint coincident L0.end L1.start
  constraint tangent L0 A0
  constraint tangent A0 L6
  measures "d210" distance of L4.start L4.end
  measures "d216" radius of A0
  measures "d228" angle of L1 L5
  measures "d232" vertical distance of L4.end L1.end
extrude "Extrude25" add sketch "Sketch24" against normal blind 20 contours L1 L4 L5 A0 L6 bodies 8
sketch "Sketch25" plane through (0, 0, -7.75) normal (0, 0, 1) x (-1, 0, 0)
  line L0 (-72.3, 0.25) -> (-72.3, -65.25)
  line L1 (-72.3, -65.25) -> (-53.3, -65.25)
  line L2 (-53.3, -65.25) -> (-53.3, 0.25)
  line L3 (-53.3, 0.25) -> (-72.3, 0.25)
  circle A0 centre (-62.55, -22.5) radius 2.5
  circle A1 centre (-62.55, -42.5) radius 2.5
  circle A2 centre (-62.55, -57.5) radius 2.5
  circle A3 centre (-62.55, -22.5) radius 2.5
  circle A4 centre (-62.55, -7.5) radius 2.5
  point P0 (-65.05, -42.5)
extrude "Extrude26" cut sketch "Sketch25" along normal through all and the other way up to surface (3 mm away) contours A0 A3 | A1 | A2 | A4 bodies 8
chamfer "Chamfer5" distance 1 angle 45 4 edges at (64.8808, 21.596, 8.25) (64.8808, 41.596, 8.25) (64.8808, 6.596, 8.25) (64.8808, 56.596, 8.25) on bodies 8
sketch "Sketch26" plane through (0, 0, 2.75) normal (0, 0, 1) x (-1, 0, 0)
  circle A0 centre (-62.55, -7.5) radius 2.5
  circle A1 centre (-62.55, -22.5) radius 2.5
  circle A2 centre (-191.6402, 133.2189) radius 1.55
  circle A3 centre (-214.9747, 133.2189) radius 1.55
  circle A4 centre (-191.6402, 156.5534) radius 1.55
  circle A5 centre (-214.9747, 156.5534) radius 1.55
  line L0 (-103.2458, -11.6764) -> (-190.8258, 108.8671)
  arc A6 (-173.1261, 121.7267) -> (-190.8258, 108.8671) centre (-181.976, 115.2969) ccw
  line L1 (-173.1261, 121.7267) -> (-85.5457, 1.1826)
  arc A7 (-87.881, -14.1099) -> (-85.5457, 1.1826) centre (-94.4449, -5.283) ccw
  arc A8 (-103.2458, -11.6764) -> (-87.881, -14.1099) centre (-94.3466, -5.2108) ccw
  line L2 (-52.55, -31.75) -> (-52.55, -2.75)
  line L3 (-52.55, -2.75) -> (-72.8, -2.75)
  line L4 (-72.8, -2.75) -> (-74.9796, 0.25)
  line L5 (-74.9796, 0.25) -> (-46.8, 0.25)
  line L6 (-46.8, 0.25) -> (-46.8, 3)
  line L7 (-46.8, 3) -> (-84.2727, 13.0408)
  line L8 (-84.2727, 13.0408) -> (-190.3571, 159.0534)
  line L9 (-190.3571, 159.0534) -> (-217.4747, 159.0534)
  line L10 (-217.4747, 159.0534) -> (-217.4747, 131.9358)
  line L11 (-217.4747, 131.9358) -> (-98.55, -31.75)
  line L12 (-98.55, -31.75) -> (-52.55, -31.75)
  line L13 (-47.9796, 3.8337) -> (-74.9796, 11.0683)
  line L14 (-47.9796, 3.8337) -> (-47.9796, 0)
  line L15 (-47.9796, 0) -> (-74.9796, 0)
  line L16 (-74.9796, 0) -> (-74.9796, 11.0683)
  line L17 (-72.3, 0) -> (22.5, 0)
  dimension "d217" = 0.5
  dimension "d218" = 27
  constraint perpendicular L5 L14
  constraint perpendicular L14 L15
  constraint coincident L13 L16.end
  constraint perpendicular L5 L16
  constraint vertical L4.end L15.end
  constraint horizontal L15.end L17.start
  constraint coincident L13.end L16.end
  measures "d218" distance of L14.end L15.end
extrude "Extrude27" cut sketch "Sketch26" along normal blind -9 and the other way blind -0.5 contours L5 L7 L14 L16 | L7 L13 L14 L16 bodies 8
extrude "Extrude28" add sketch "Sketch24" along normal blind 17 from surface at -80.5 contours L1 L4 L5 A0 L6 bodies 8
sketch "Battery" plane through (0, 68.25, 0) normal (0, 1, 0) x (-1, 0, 0)
  line L0 (-38.4, -46.861) -> (-11.4, -46.861)
  line L1 (-11.4, -46.861) -> (-11.4, -89.861)
  line L2 (-11.4, -89.861) -> (-38.4, -89.861)
  line L3 (-38.4, -89.861) -> (-38.4, -46.861)
  line L4 (-24.9, -46.861) -> (-24.9, -4)
  line L5 (-2.9686, -4) -> (-46.8314, -4)
  dimension "d226" = 43
  dimension "d227" = 27
  constraint horizontal L0
  constraint vertical L1
  constraint horizontal L2
  constraint vertical L3
  constraint midpoint L0 L4.start
  constraint perpendicular L0 L4
  constraint midpoint L4.end L5
  measures "d226" distance of L0.end L1.end
  measures "d227" distance of L1.end L2.end
sketch "Sketch28" plane through (0, 68.25, 0) normal (0, 1, 0) x (-1, 0, 0)
  line L0 (-40.6513, -100.75) -> (-53.3, -10.75)
  line L1 (-41.7757, -92.75) -> (-25.4, -92.75)
  line L2 (-25.4, -92.75) -> (-25.4, -100.75)
  line L3 (-25.4, -100.75) -> (-40.6513, -100.75)
  line L4 (-2.9686, -4) -> (-46.8314, -4)
  line L5 (-24.9, -4) -> (-24.9, -92)
  dimension "d229" = 8
  dimension "d230" = 88
  dimension "d231" = 0.5
  constraint coincident L0 L1.start
  constraint horizontal L1
  constraint coincident L0.start L3.end
  constraint horizontal L3
  constraint vertical L2
  constraint midpoint L4 L5.start
  constraint perpendicular L4 L5
  measures "d229" distance of L1.end L2.end
  measures "d230" distance of L5.start L5.end
  measures "d231" distance of L2 L5
extrude "Extrude29" add sketch "Sketch28" against normal blind 80.5 bodies 8
fillet "Fillet5" radius 7 2 edges at (41.7757, 58.25, -92.75) (41.7757, -3.75, -92.75) on bodies 8
sketch "Sketch29" plane through (0, 0, -100.75) normal (0, 0, -1) x (1, 0, 0)
  line L0 (50.6513, 12.25) -> (25.4, 12.25)
  line L1 (25.4, 12.25) -> (25.4, -68.25)
  line L2 (25.4, -68.25) -> (50.6513, -68.25)
  line L3 (50.6513, -68.25) -> (50.6513, -48.25)
  line L4 (50.6513, -48.25) -> (40.6513, -48.25)
  line L5 (40.6513, -48.25) -> (40.6513, -4.75)
  line L6 (40.6513, -4.75) -> (50.6513, -4.75)
  line L7 (50.6513, -4.75) -> (50.6513, 12.25)
  line L8 (52.6513, -48.25) -> (40.6513, -26.5)
  line L9 (52.6513, -4.75) -> (40.6513, -26.5)
  line L10 (50.6513, -48.25) -> (70.7046, -48.25)
  line L11 (70.7046, -4.75) -> (50.6513, -4.75)
  dimension "d240" = 12
  dimension "d243" = 28.887
  constraint midpoint L5 L8.end
  constraint coincident L8.start L10
  constraint vertical L8.start L9.start
  constraint coincident L9.start L11
  measures "d240" distance of L4.end L8.start
  measures "d243" angle of L5 L9
extrude "Extrude30" add sketch "Sketch29" against normal blind 8 contours L5 L6 L9 L11 | L4 L5 L8 L10 bodies 8
extrude "Extrude31" cut 1 faces at (51.9847, 48.25, -98.1745) along direction (0, 1, 0) through all and the other way through all on bodies 8 bodies 8
mirror "Mirror2" about plane through (24.9, 37.5, 5) normal (-1, 0, 0) of bodies 8 makes body 9
move_body "Move3" bodies 3 5 to x (1, 0, 0) y (0, 1, 0) z (0, 0, 1) at (0, 0, -1.25)
equation "d116 = ( 19.5 / 2 ) * 1 mm"
equation "d126 = ( ( 12.5 mm - d105 ) / 2 )"
equation "d192 = ( 4.8 / 2 ) * 1 mm"
named bodies: "Main Body", "Rear Left", "Front Right", "Rear Right", "Front Left", "Camera Holder", "Pin", "Battery Holder Right", "Battery Holder Left"
